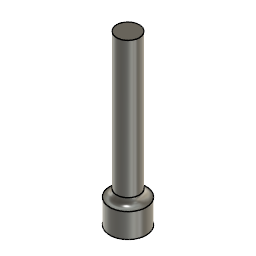
rod0406 (Autodesk Fusion 360 design; units mm, degrees)
Autodesk Fusion 360 part; units mm, degrees
sketch "Sketch1" plane through (0, 0, 0) normal (0, 0, 1) x (1, 0, 0)
  circle A0 centre (0, 0) radius 3.75
  line L0 (-1.6, 0, 50) -> (-1.6, 2.1749, 50)
  line L1 (1.6, 0, 50) -> (1.6, 2.1749, 50)
  line L2 (-1.6, 0, 50) -> (-1.6, -2.1749, 50)
  circle A1 through (6, 0, 50) (-3, 5.1962, 50) (-3, -5.1962, 50)
  line L3 (1.6, 0, 50) -> (1.6, -2.1749, 50)
  line L4 (1.5, 0, 50) -> (1.6, 0, 50)
  circle A2 through (2.7, 0, 50) (-1.35, 2.3383, 50) (-1.35, -2.3383, 50)
  circle A3 through (3.75, 0, 50) (-1.875, 3.2476, 50) (-1.875, -3.2476, 50)
  dimension "d1" = 7.5
  dimension "d4" = 1.5
  dimension "d5" = 5.4
  dimension "d6" = 1.6
  dimension "d7" = 12
  dimension "d8" = 7.5
  constraint coincident A0.centre origin
  measures "d1" diameter of A0
extrude "Extrude1" add sketch "Sketch1" along normal blind 50
extrude "Extrude2" add sketch "Sketch1" against normal blind 8 contours A1 in plane through (0, 0, 50) normal (0, 0, 1)
fillet "Fillet1" radius 2.4 1 edges at (-3.4962, 1.3561, 42)
extrude "Extrude3" cut sketch "Sketch1" against normal blind 6 contours L0 L1 L2 L3 A2 in plane through (0, 0, 50) normal (0, 0, 1)
move_body "Move1" bodies 1 to x (1, 0, 0) y (0, -1, 0) z (0, 0, -1) at (0.0488, -2.4837, 50.0384)
move_face "OffsetFaces1" offset 5.4 1 faces at (0.938, -3.1049, 50.0384)
